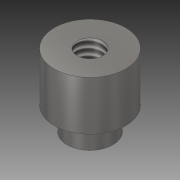
# Autodesk Inventor part: Spacer M2 3mm
Saved by Autodesk Inventor 2019.1 (Build 231200000, 200)
## iProperties
Part Number: Spacer M2 3mm
Material: Stahl, weich
Document SubType Name: Modeling
Designer: rYan
Mass: 0.351052 g
Surface Area: 1.0084 cm^2
Volume: 0.0447201 cm^3
Density: 7.85 g/cm^3
Appearance: Halbpoliert
Author: rYan
Autodesk Inventor part; units mm, degrees
ref_plane "YZ Plane" through (0, 0, 0) normal (1, 0, 0) x (0, 1, 0)
ref_plane "XZ Plane" through (0, 0, 0) normal (0, 1, 0) x (-1, 0, 0)
ref_plane "XY Plane" through (0, 0, 0) normal (0, 0, 1) x (1, 0, 0)
sketch "Skizze1" plane through (0, 0, 0) normal (0, 1, 0) x (-1, 0, 0)
  line L0 (0, 0) -> (0, 4.4)
  line L1 (0, 4.4) -> (-2.175, 4.4)
  line L2 (-2.175, 4.4) -> (-2.175, 1.4)
  line L3 (-2.175, 1.4) -> (-1.4, 1.4)
  line L4 (-1.4, 1.4) -> (-1.4, 0)
  line L5 (-1.4, 0) -> (0, 0)
  dimension "d0" = 4.35
  dimension "d1" = 1.4
  dimension "d2" = 3
  dimension "d3" = 2.8
  constraints: 12 end point, 5 perpendicular, 1 vertical
  measures "d0" diameter of L2 L0
  measures "d1" distance between parallel lines of L5 L3
  measures "d2" distance between parallel lines of L3 L1
  measures "d3" diameter of L4 L0
revolve "Umdrehung1" add sketch "Skizze1" angle 360 about axis through (0, 0, 0) along (0, 0, 1)
sketch "Skizze2" plane through (0, 0, 4.4) normal (0, 0, 1) x (1, 0, 0)
  point P0 (0, 0)
  point P1 (0, 0)
  constraints: 1 coincident
hole "Bohrung1" at (0, 0, 4.4) direction (0, 0, -1) diameter 1.567 end through all thread size "M2x0.4" class "6H" standard "ISO Metric profile"
